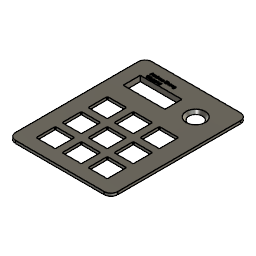
Case Top (Autodesk Fusion 360 design; units mm, degrees)
part number: 2026-02-07-01-16-41-371
Autodesk Fusion 360 part; units mm, degrees
sketch "plate-2026-02-07T04_57_06.028Z" plane through (0, 0, 0) normal (0, 0, 1) x (1, 0, 0)
  line L0 (3.025, -21.575) -> (16.025, -21.575)
  line L1 (3.025, -35.575) -> (16.025, -35.575)
  line L2 (2.525, -22.075) -> (2.525, -35.075)
  line L3 (16.525, -22.075) -> (16.525, -35.075)
  arc A0 (3.025, -21.575) -> (2.525, -22.075) centre (3.025, -22.075) ccw
  arc A1 (16.525, -22.075) -> (16.025, -21.575) centre (16.025, -22.075) ccw
  arc A2 (2.525, -35.075) -> (3.025, -35.575) centre (3.025, -35.075) ccw
  arc A3 (16.025, -35.575) -> (16.525, -35.075) centre (16.025, -35.075) ccw
  line L4 (22.075, -21.575) -> (35.075, -21.575)
  line L5 (22.075, -35.575) -> (35.075, -35.575)
  line L6 (21.575, -22.075) -> (21.575, -35.075)
  line L7 (35.575, -22.075) -> (35.575, -35.075)
  arc A4 (22.075, -21.575) -> (21.575, -22.075) centre (22.075, -22.075) ccw
  arc A5 (35.575, -22.075) -> (35.075, -21.575) centre (35.075, -22.075) ccw
  arc A6 (21.575, -35.075) -> (22.075, -35.575) centre (22.075, -35.075) ccw
  arc A7 (35.075, -35.575) -> (35.575, -35.075) centre (35.075, -35.075) ccw
  line L8 (41.125, -21.575) -> (54.125, -21.575)
  line L9 (41.125, -35.575) -> (54.125, -35.575)
  line L10 (40.625, -22.075) -> (40.625, -35.075)
  line L11 (54.625, -22.075) -> (54.625, -35.075)
  arc A8 (41.125, -21.575) -> (40.625, -22.075) centre (41.125, -22.075) ccw
  arc A9 (54.625, -22.075) -> (54.125, -21.575) centre (54.125, -22.075) ccw
  arc A10 (40.625, -35.075) -> (41.125, -35.575) centre (41.125, -35.075) ccw
  arc A11 (54.125, -35.575) -> (54.625, -35.075) centre (54.125, -35.075) ccw
  line L12 (3.025, -40.625) -> (16.025, -40.625)
  line L13 (3.025, -54.625) -> (16.025, -54.625)
  line L14 (2.525, -41.125) -> (2.525, -54.125)
  line L15 (16.525, -41.125) -> (16.525, -54.125)
  arc A12 (3.025, -40.625) -> (2.525, -41.125) centre (3.025, -41.125) ccw
  arc A13 (16.525, -41.125) -> (16.025, -40.625) centre (16.025, -41.125) ccw
  arc A14 (2.525, -54.125) -> (3.025, -54.625) centre (3.025, -54.125) ccw
  arc A15 (16.025, -54.625) -> (16.525, -54.125) centre (16.025, -54.125) ccw
  line L16 (22.075, -40.625) -> (35.075, -40.625)
  line L17 (22.075, -54.625) -> (35.075, -54.625)
  line L18 (21.575, -41.125) -> (21.575, -54.125)
  line L19 (35.575, -41.125) -> (35.575, -54.125)
  arc A16 (22.075, -40.625) -> (21.575, -41.125) centre (22.075, -41.125) ccw
  arc A17 (35.575, -41.125) -> (35.075, -40.625) centre (35.075, -41.125) ccw
  arc A18 (21.575, -54.125) -> (22.075, -54.625) centre (22.075, -54.125) ccw
  arc A19 (35.075, -54.625) -> (35.575, -54.125) centre (35.075, -54.125) ccw
  line L20 (41.125, -40.625) -> (54.125, -40.625)
  line L21 (41.125, -54.625) -> (54.125, -54.625)
  line L22 (40.625, -41.125) -> (40.625, -54.125)
  line L23 (54.625, -41.125) -> (54.625, -54.125)
  arc A20 (41.125, -40.625) -> (40.625, -41.125) centre (41.125, -41.125) ccw
  arc A21 (54.625, -41.125) -> (54.125, -40.625) centre (54.125, -41.125) ccw
  arc A22 (40.625, -54.125) -> (41.125, -54.625) centre (41.125, -54.125) ccw
  arc A23 (54.125, -54.625) -> (54.625, -54.125) centre (54.125, -54.125) ccw
  line L24 (3.025, -59.675) -> (16.025, -59.675)
  line L25 (3.025, -73.675) -> (16.025, -73.675)
  line L26 (2.525, -60.175) -> (2.525, -73.175)
  line L27 (16.525, -60.175) -> (16.525, -73.175)
  arc A24 (3.025, -59.675) -> (2.525, -60.175) centre (3.025, -60.175) ccw
  arc A25 (16.525, -60.175) -> (16.025, -59.675) centre (16.025, -60.175) ccw
  arc A26 (2.525, -73.175) -> (3.025, -73.675) centre (3.025, -73.175) ccw
  arc A27 (16.025, -73.675) -> (16.525, -73.175) centre (16.025, -73.175) ccw
  line L28 (22.075, -59.675) -> (35.075, -59.675)
  line L29 (22.075, -73.675) -> (35.075, -73.675)
  line L30 (21.575, -60.175) -> (21.575, -73.175)
  line L31 (35.575, -60.175) -> (35.575, -73.175)
  arc A28 (22.075, -59.675) -> (21.575, -60.175) centre (22.075, -60.175) ccw
  arc A29 (35.575, -60.175) -> (35.075, -59.675) centre (35.075, -60.175) ccw
  arc A30 (21.575, -73.175) -> (22.075, -73.675) centre (22.075, -73.175) ccw
  arc A31 (35.075, -73.675) -> (35.575, -73.175) centre (35.075, -73.175) ccw
  line L32 (41.125, -59.675) -> (54.125, -59.675)
  line L33 (41.125, -73.675) -> (54.125, -73.675)
  line L34 (40.625, -60.175) -> (40.625, -73.175)
  line L35 (54.625, -60.175) -> (54.625, -73.175)
  arc A32 (41.125, -59.675) -> (40.625, -60.175) centre (41.125, -60.175) ccw
  arc A33 (54.625, -60.175) -> (54.125, -59.675) centre (54.125, -60.175) ccw
  arc A34 (40.625, -73.175) -> (41.125, -73.675) centre (41.125, -73.175) ccw
  arc A35 (54.125, -73.675) -> (54.625, -73.175) centre (54.125, -73.175) ccw
  line L36 (0, -76.2) -> (57.15, -76.2)
  line L37 (0, -19.05) -> (57.15, -19.05)
  line L38 (0, -76.2) -> (0, -19.05)
  line L39 (57.15, -76.2) -> (57.15, -19.05)
  line L40 (-8.35, -83.05) -> (66.65, -83.05)
  line L41 (66.65, -83.05) -> (66.65, 16.95)
  line L42 (66.65, 16.95) -> (-8.35, 16.95)
  line L43 (-8.35, 16.95) -> (-8.35, -83.05)
  dimension "d5" = 100
  dimension "d6" = 75
  dimension "d7" = 9.5
  dimension "d8" = 36
  constraint horizontal L40
  constraint vertical L41
  constraint horizontal L42
  constraint vertical L43
  measures "d5" distance of L40.end L41.end
  measures "d6" distance of L40.start L40.end
  measures "d7" distance of L39 L41
  measures "d8" distance of L37 L42
extrude "Extrude1" add sketch "plate-2026-02-07T04_57_06.028Z" along normal blind 2 contours L36 L37 L38 L39 | L40 L41 L42 L43
fillet "Fillet2" radius 5 4 edges at (-8.35, -83.05, 1) (66.65, -83.05, 1) (66.65, 16.95, 1) (-8.35, 16.95, 1)
sketch "Sketch3" plane through (0, 0, 2) normal (0, 0, 1) x (-1, 0, 0)
  arc A0 (3.35, -16.95) -> (8.35, -11.95) centre (3.35, -11.95) ccw
  line L0 (8.35, -11.95) -> (8.35, 78.05)
  arc A1 (8.35, 78.05) -> (3.35, 83.05) centre (3.35, 78.05) ccw
  line L1 (3.35, 83.05) -> (-61.65, 83.05)
  arc A2 (-61.65, 83.05) -> (-66.65, 78.05) centre (-61.65, 78.05) ccw
  line L2 (-66.65, 78.05) -> (-66.65, -11.95)
  arc A3 (-66.65, -11.95) -> (-61.65, -16.95) centre (-61.65, -11.95) ccw
  line L3 (-61.65, -16.95) -> (3.35, -16.95)
  arc A4 (-41.125, 21.575) -> (-40.625, 22.075) centre (-41.125, 22.075) ccw
  line L4 (-41.125, 21.575) -> (-54.125, 21.575)
  arc A5 (-54.625, 22.075) -> (-54.125, 21.575) centre (-54.125, 22.075) ccw
  line L5 (-54.625, 22.075) -> (-54.625, 35.075)
  arc A6 (-54.125, 35.575) -> (-54.625, 35.075) centre (-54.125, 35.075) ccw
  line L6 (-54.125, 35.575) -> (-41.125, 35.575)
  arc A7 (-40.625, 35.075) -> (-41.125, 35.575) centre (-41.125, 35.075) ccw
  line L7 (-40.625, 35.075) -> (-40.625, 22.075)
  arc A8 (-22.075, 21.575) -> (-21.575, 22.075) centre (-22.075, 22.075) ccw
  line L8 (-22.075, 21.575) -> (-35.075, 21.575)
  arc A9 (-35.575, 22.075) -> (-35.075, 21.575) centre (-35.075, 22.075) ccw
  line L9 (-35.575, 22.075) -> (-35.575, 35.075)
  arc A10 (-35.075, 35.575) -> (-35.575, 35.075) centre (-35.075, 35.075) ccw
  line L10 (-35.075, 35.575) -> (-22.075, 35.575)
  arc A11 (-21.575, 35.075) -> (-22.075, 35.575) centre (-22.075, 35.075) ccw
  line L11 (-21.575, 35.075) -> (-21.575, 22.075)
  arc A12 (-3.025, 59.675) -> (-2.525, 60.175) centre (-3.025, 60.175) ccw
  line L12 (-3.025, 59.675) -> (-16.025, 59.675)
  arc A13 (-16.525, 60.175) -> (-16.025, 59.675) centre (-16.025, 60.175) ccw
  line L13 (-16.525, 60.175) -> (-16.525, 73.175)
  arc A14 (-16.025, 73.675) -> (-16.525, 73.175) centre (-16.025, 73.175) ccw
  line L14 (-16.025, 73.675) -> (-3.025, 73.675)
  arc A15 (-2.525, 73.175) -> (-3.025, 73.675) centre (-3.025, 73.175) ccw
  line L15 (-2.525, 73.175) -> (-2.525, 60.175)
  arc A16 (-22.075, 40.625) -> (-21.575, 41.125) centre (-22.075, 41.125) ccw
  line L16 (-22.075, 40.625) -> (-35.075, 40.625)
  arc A17 (-35.575, 41.125) -> (-35.075, 40.625) centre (-35.075, 41.125) ccw
  line L17 (-35.575, 41.125) -> (-35.575, 54.125)
  arc A18 (-35.075, 54.625) -> (-35.575, 54.125) centre (-35.075, 54.125) ccw
  line L18 (-35.075, 54.625) -> (-22.075, 54.625)
  arc A19 (-21.575, 54.125) -> (-22.075, 54.625) centre (-22.075, 54.125) ccw
  line L19 (-21.575, 54.125) -> (-21.575, 41.125)
  arc A20 (-3.025, 40.625) -> (-2.525, 41.125) centre (-3.025, 41.125) ccw
  line L20 (-3.025, 40.625) -> (-16.025, 40.625)
  arc A21 (-16.525, 41.125) -> (-16.025, 40.625) centre (-16.025, 41.125) ccw
  line L21 (-16.525, 41.125) -> (-16.525, 54.125)
  arc A22 (-16.025, 54.625) -> (-16.525, 54.125) centre (-16.025, 54.125) ccw
  line L22 (-16.025, 54.625) -> (-3.025, 54.625)
  arc A23 (-2.525, 54.125) -> (-3.025, 54.625) centre (-3.025, 54.125) ccw
  line L23 (-2.525, 54.125) -> (-2.525, 41.125)
  arc A24 (-41.125, 59.675) -> (-40.625, 60.175) centre (-41.125, 60.175) ccw
  line L24 (-41.125, 59.675) -> (-54.125, 59.675)
  arc A25 (-54.625, 60.175) -> (-54.125, 59.675) centre (-54.125, 60.175) ccw
  line L25 (-54.625, 60.175) -> (-54.625, 73.175)
  arc A26 (-54.125, 73.675) -> (-54.625, 73.175) centre (-54.125, 73.175) ccw
  line L26 (-54.125, 73.675) -> (-41.125, 73.675)
  arc A27 (-40.625, 73.175) -> (-41.125, 73.675) centre (-41.125, 73.175) ccw
  line L27 (-40.625, 73.175) -> (-40.625, 60.175)
  arc A28 (-22.075, 59.675) -> (-21.575, 60.175) centre (-22.075, 60.175) ccw
  line L28 (-22.075, 59.675) -> (-35.075, 59.675)
  arc A29 (-35.575, 60.175) -> (-35.075, 59.675) centre (-35.075, 60.175) ccw
  line L29 (-35.575, 60.175) -> (-35.575, 73.175)
  arc A30 (-35.075, 73.675) -> (-35.575, 73.175) centre (-35.075, 73.175) ccw
  line L30 (-35.075, 73.675) -> (-22.075, 73.675)
  arc A31 (-21.575, 73.175) -> (-22.075, 73.675) centre (-22.075, 73.175) ccw
  line L31 (-21.575, 73.175) -> (-21.575, 60.175)
  arc A32 (-3.025, 21.575) -> (-2.525, 22.075) centre (-3.025, 22.075) ccw
  line L32 (-3.025, 21.575) -> (-16.025, 21.575)
  arc A33 (-16.525, 22.075) -> (-16.025, 21.575) centre (-16.025, 22.075) ccw
  line L33 (-16.525, 22.075) -> (-16.525, 35.075)
  arc A34 (-16.025, 35.575) -> (-16.525, 35.075) centre (-16.025, 35.075) ccw
  line L34 (-16.025, 35.575) -> (-3.025, 35.575)
  arc A35 (-2.525, 35.075) -> (-3.025, 35.575) centre (-3.025, 35.075) ccw
  line L35 (-2.525, 35.075) -> (-2.525, 22.075)
  arc A36 (-41.125, 40.625) -> (-40.625, 41.125) centre (-41.125, 41.125) ccw
  line L36 (-41.125, 40.625) -> (-54.125, 40.625)
  arc A37 (-54.625, 41.125) -> (-54.125, 40.625) centre (-54.125, 41.125) ccw
  line L37 (-54.625, 41.125) -> (-54.625, 54.125)
  arc A38 (-54.125, 54.625) -> (-54.625, 54.125) centre (-54.125, 54.125) ccw
  line L38 (-54.125, 54.625) -> (-41.125, 54.625)
  arc A39 (-40.625, 54.125) -> (-41.125, 54.625) centre (-41.125, 54.125) ccw
  line L39 (-40.625, 54.125) -> (-40.625, 41.125)
  circle A40 centre (-47.85, 2.15) radius 5
  line L40 (-3.15, -1.95) -> (-29.65, -1.95)
  line L41 (-29.65, -1.95) -> (-29.65, 6.55)
  line L42 (-29.65, 6.55) -> (-3.15, 6.55)
  line L43 (-3.15, 6.55) -> (-3.15, -1.95)
  dimension "d17" = 10
  dimension "d18" = 18.8
  dimension "d19" = 19.1
  dimension "d22" = 15
  dimension "d23" = 26.5
  dimension "d24" = 11.5
  dimension "d25" = 8.5
  constraint horizontal L40
  constraint vertical L41
  constraint horizontal L42
  constraint vertical L43
  measures "d17" diameter of A40
  measures "d18" distance of L2 A40.centre
  measures "d19" distance of L3 A40.centre
  measures "d22" distance of L3 L40
  measures "d23" distance of L41 L43
  measures "d24" distance of L0 L43
  measures "d25" distance of L40 L42
extrude "Extrude2" cut sketch "Sketch3" against normal up to surface (2 mm away) contours A40 | L40 L41 L42 L43
chamfer "Chamfer1" distance 2 angle 45 5 edges at (16.4, 1.95, 2) (29.65, -2.3, 2) (3.15, -2.3, 2) (16.4, -6.55, 2) (52.5116, -3.9581, 2)
sketch "Sketch4" plane through (0, 0, 2) normal (0, 0, 1) x (-1, 0, 0)
  line L0 (-31.65, 8.55) -> (-1.15, 8.55)
  line L1 (-1.15, 8.55) -> (-1.15, -3.95)
  line L2 (-1.15, -3.95) -> (-31.65, -3.95)
  line L3 (-31.65, -3.95) -> (-31.65, 8.55)
  arc A0 (3.35, -16.95) -> (8.35, -11.95) centre (3.35, -11.95) ccw
  line L4 (8.35, -11.95) -> (8.35, 78.05)
  arc A1 (8.35, 78.05) -> (3.35, 83.05) centre (3.35, 78.05) ccw
  line L5 (3.35, 83.05) -> (-61.65, 83.05)
  arc A2 (-61.65, 83.05) -> (-66.65, 78.05) centre (-61.65, 78.05) ccw
  line L6 (-66.65, 78.05) -> (-66.65, -11.95)
  arc A3 (-66.65, -11.95) -> (-61.65, -16.95) centre (-61.65, -11.95) ccw
  line L7 (-61.65, -16.95) -> (3.35, -16.95)
  arc A4 (-3.025, 21.575) -> (-2.525, 22.075) centre (-3.025, 22.075) ccw
  line L8 (-3.025, 21.575) -> (-16.025, 21.575)
  arc A5 (-16.525, 22.075) -> (-16.025, 21.575) centre (-16.025, 22.075) ccw
  line L9 (-16.525, 22.075) -> (-16.525, 35.075)
  arc A6 (-16.025, 35.575) -> (-16.525, 35.075) centre (-16.025, 35.075) ccw
  line L10 (-16.025, 35.575) -> (-3.025, 35.575)
  arc A7 (-2.525, 35.075) -> (-3.025, 35.575) centre (-3.025, 35.075) ccw
  line L11 (-2.525, 35.075) -> (-2.525, 22.075)
  arc A8 (-41.125, 59.675) -> (-40.625, 60.175) centre (-41.125, 60.175) ccw
  line L12 (-41.125, 59.675) -> (-54.125, 59.675)
  arc A9 (-54.625, 60.175) -> (-54.125, 59.675) centre (-54.125, 60.175) ccw
  line L13 (-54.625, 60.175) -> (-54.625, 73.175)
  arc A10 (-54.125, 73.675) -> (-54.625, 73.175) centre (-54.125, 73.175) ccw
  line L14 (-54.125, 73.675) -> (-41.125, 73.675)
  arc A11 (-40.625, 73.175) -> (-41.125, 73.675) centre (-41.125, 73.175) ccw
  line L15 (-40.625, 73.175) -> (-40.625, 60.175)
  arc A12 (-22.075, 59.675) -> (-21.575, 60.175) centre (-22.075, 60.175) ccw
  line L16 (-22.075, 59.675) -> (-35.075, 59.675)
  arc A13 (-35.575, 60.175) -> (-35.075, 59.675) centre (-35.075, 60.175) ccw
  line L17 (-35.575, 60.175) -> (-35.575, 73.175)
  arc A14 (-35.075, 73.675) -> (-35.575, 73.175) centre (-35.075, 73.175) ccw
  line L18 (-35.075, 73.675) -> (-22.075, 73.675)
  arc A15 (-21.575, 73.175) -> (-22.075, 73.675) centre (-22.075, 73.175) ccw
  line L19 (-21.575, 73.175) -> (-21.575, 60.175)
  arc A16 (-22.075, 40.625) -> (-21.575, 41.125) centre (-22.075, 41.125) ccw
  line L20 (-22.075, 40.625) -> (-35.075, 40.625)
  arc A17 (-35.575, 41.125) -> (-35.075, 40.625) centre (-35.075, 41.125) ccw
  line L21 (-35.575, 41.125) -> (-35.575, 54.125)
  arc A18 (-35.075, 54.625) -> (-35.575, 54.125) centre (-35.075, 54.125) ccw
  line L22 (-35.075, 54.625) -> (-22.075, 54.625)
  arc A19 (-21.575, 54.125) -> (-22.075, 54.625) centre (-22.075, 54.125) ccw
  line L23 (-21.575, 54.125) -> (-21.575, 41.125)
  arc A20 (-3.025, 59.675) -> (-2.525, 60.175) centre (-3.025, 60.175) ccw
  line L24 (-3.025, 59.675) -> (-16.025, 59.675)
  arc A21 (-16.525, 60.175) -> (-16.025, 59.675) centre (-16.025, 60.175) ccw
  line L25 (-16.525, 60.175) -> (-16.525, 73.175)
  arc A22 (-16.025, 73.675) -> (-16.525, 73.175) centre (-16.025, 73.175) ccw
  line L26 (-16.025, 73.675) -> (-3.025, 73.675)
  arc A23 (-2.525, 73.175) -> (-3.025, 73.675) centre (-3.025, 73.175) ccw
  line L27 (-2.525, 73.175) -> (-2.525, 60.175)
  arc A24 (-41.125, 40.625) -> (-40.625, 41.125) centre (-41.125, 41.125) ccw
  line L28 (-41.125, 40.625) -> (-54.125, 40.625)
  arc A25 (-54.625, 41.125) -> (-54.125, 40.625) centre (-54.125, 41.125) ccw
  line L29 (-54.625, 41.125) -> (-54.625, 54.125)
  arc A26 (-54.125, 54.625) -> (-54.625, 54.125) centre (-54.125, 54.125) ccw
  line L30 (-54.125, 54.625) -> (-41.125, 54.625)
  arc A27 (-40.625, 54.125) -> (-41.125, 54.625) centre (-41.125, 54.125) ccw
  line L31 (-40.625, 54.125) -> (-40.625, 41.125)
  arc A28 (-3.025, 40.625) -> (-2.525, 41.125) centre (-3.025, 41.125) ccw
  line L32 (-3.025, 40.625) -> (-16.025, 40.625)
  arc A29 (-16.525, 41.125) -> (-16.025, 40.625) centre (-16.025, 41.125) ccw
  line L33 (-16.525, 41.125) -> (-16.525, 54.125)
  arc A30 (-16.025, 54.625) -> (-16.525, 54.125) centre (-16.025, 54.125) ccw
  line L34 (-16.025, 54.625) -> (-3.025, 54.625)
  arc A31 (-2.525, 54.125) -> (-3.025, 54.625) centre (-3.025, 54.125) ccw
  line L35 (-2.525, 54.125) -> (-2.525, 41.125)
  arc A32 (-22.075, 21.575) -> (-21.575, 22.075) centre (-22.075, 22.075) ccw
  line L36 (-22.075, 21.575) -> (-35.075, 21.575)
  arc A33 (-35.575, 22.075) -> (-35.075, 21.575) centre (-35.075, 22.075) ccw
  line L37 (-35.575, 22.075) -> (-35.575, 35.075)
  arc A34 (-35.075, 35.575) -> (-35.575, 35.075) centre (-35.075, 35.075) ccw
  line L38 (-35.075, 35.575) -> (-22.075, 35.575)
  arc A35 (-21.575, 35.075) -> (-22.075, 35.575) centre (-22.075, 35.075) ccw
  line L39 (-21.575, 35.075) -> (-21.575, 22.075)
  arc A36 (-41.125, 21.575) -> (-40.625, 22.075) centre (-41.125, 22.075) ccw
  line L40 (-41.125, 21.575) -> (-54.125, 21.575)
  arc A37 (-54.625, 22.075) -> (-54.125, 21.575) centre (-54.125, 22.075) ccw
  line L41 (-54.625, 22.075) -> (-54.625, 35.075)
  arc A38 (-54.125, 35.575) -> (-54.625, 35.075) centre (-54.125, 35.075) ccw
  line L42 (-54.125, 35.575) -> (-41.125, 35.575)
  arc A39 (-40.625, 35.075) -> (-41.125, 35.575) centre (-41.125, 35.075) ccw
  line L43 (-40.625, 35.075) -> (-40.625, 22.075)
  circle A40 centre (-47.85, 2.15) radius 7
  line L44 (-4, -3.952) -> (-31.65, -3.95) construction
  line L45 (-31.65, -3.95) -> (-31.6504, -10) construction
  line L46 (-31.6504, -10) -> (-4.0004, -10.002) construction
  line L47 (-4.0004, -10.002) -> (-4, -3.952) construction
  dimension "d27" = 2
  text T0 "Andrew Zhang  Gigapad" font "Arial" height 2 align left top in box 27.65 x 6.05 at (-4, -3.952) x (-1, 0.000071) y (-0.000071, -1) spacing 1 kerned
  constraint coincident L2.end
emboss "Emboss1" depth 0.2 profiles "Sketch4" section 1 text T0 onto face at (29.9832, 12.6165, 2)
equation "d28 = 'Andrew Zhang  Gigapad'"
